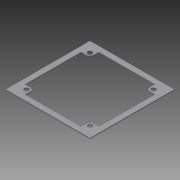
# Autodesk Inventor part: DistancePlate
Saved by Autodesk Inventor 2015 (Build 190159000, 159)
## iProperties
Created: 2022-04-22
Part Number: DistancePlate
Material: Generic
Document SubType Name: Modeling
Designer: Jan
Density: 1 g/cm^3
Appearance: Default
Author: Jan
Autodesk Inventor part; units mm, degrees
ref_plane "YZ Plane" through (0, 0, 0) normal (1, 0, 0) x (0, 1, 0)
ref_plane "XZ Plane" through (0, 0, 0) normal (0, 1, 0) x (-1, 0, 0)
ref_plane "XY Plane" through (0, 0, 0) normal (0, 0, 1) x (1, 0, 0)
sketch "Sketch1" plane through (0, 0, 0) normal (0, 0, 1) x (1, 0, 0)
  line L0 (-24.8, 24.8) -> (24.8, 24.8)
  line L1 (24.8, 24.8) -> (24.8, -24.8)
  line L2 (24.8, -24.8) -> (-24.8, -24.8)
  line L3 (-24.8, -24.8) -> (-24.8, 24.8)
  line L4 (-16.6, 21.8) -> (16.6, 21.8)
  line L5 (21.8, 16.6) -> (21.8, -16.6)
  line L6 (16.6, -21.8) -> (-16.6, -21.8)
  line L7 (-21.8, -16.6) -> (-21.8, 16.6)
  arc A0 (-18.75, 16.6) -> (-16.6, 18.75) centre (-18.75, 18.75) ccw
  arc A1 (-16.6, -18.75) -> (-18.75, -16.6) centre (-18.75, -18.75) ccw
  arc A2 (18.75, -16.6) -> (16.6, -18.75) centre (18.75, -18.75) ccw
  arc A3 (16.6, 18.75) -> (18.75, 16.6) centre (18.75, 18.75) ccw
  line L8 (-16.6, -18.75) -> (-16.6, -21.8)
  line L9 (-18.75, -16.6) -> (-21.8, -16.6)
  line L10 (-18.75, 16.6) -> (-21.8, 16.6)
  line L11 (-16.6, 18.75) -> (-16.6, 21.8)
  line L12 (18.75, 16.6) -> (21.8, 16.6)
  line L13 (16.6, 18.75) -> (16.6, 21.8)
  line L14 (18.75, -16.6) -> (21.8, -16.6)
  line L15 (16.6, -18.75) -> (16.6, -21.8)
  line L16 (0, 34.72) -> (0, -34.72) projected
  line L17 (-34.72, 0) -> (34.72, 0) projected
  circle A4 centre (-18.75, 18.75) radius 1.4
  circle A5 centre (18.75, 18.75) radius 1.4
  circle A6 centre (18.75, -18.75) radius 1.4
  circle A7 centre (-18.75, -18.75) radius 1.4
  point P0 (0, 0)
  dimension "d0" = 37.5
  dimension "d2" = 37.5
  dimension "d3" = 5.2
  dimension "d4" = 2.8
  dimension "d5" = 43.6
  dimension "d6" = 3
  dimension "d7" = 3
  dimension "d8" = 3
  dimension "d9" = 3
  constraints: 32 end point, 13 perpendicular, 8 centre point, 8 point on circle, 8 tangent, 4 coincident, 4 collinear, 4 parallel, 3 equal radius, 2 horizontal, 2 horizontal alignment, 2 vertical alignment, 2 other
  measures "d0" distance of A3.centre A0.centre
  measures "d2" distance of A2.centre A3.centre
  measures "d3" distance between parallel lines of L13 L5
  measures "d4" diameter of A4
  measures "d5" distance between parallel lines of L5 L7
  measures "d6" distance between parallel lines of L3 L7
  measures "d7" distance between parallel lines of L0 L4
  measures "d8" distance between parallel lines of L1 L5
  measures "d9" distance between parallel lines of L2 L6
extrude "Extrusion1" add sketch "Sketch1" along normal blind 0.6 contours L0 L16 L4 L11 A0 L10 L7 L17 L3 | L0 L1 L17 L5 L12 A3 L13 L4 L16 | L17 L7 L9 A1 L8 L6 L16 L2 L3 | L1 L2 L16 L6 L15 A2 L14 L5 L17
body "Solid1"
